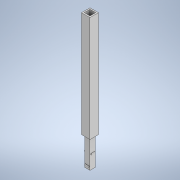
# Autodesk Inventor part: Część1
Saved by Autodesk Inventor 2022 (Build 260153000, 153)
## iProperties
Created: 2022-10-22
Part Number: Część1
Material: Ogólny
Document SubType Name: Modeling
Designer: kosak
Density: 1 g/cm^3
Appearance: Domyślna
Author: kosak
Autodesk Inventor part; units mm, degrees
ref_plane "YZ Plane" through (0, 0, 0) normal (1, 0, 0) x (0, 1, 0)
ref_plane "XZ Plane" through (0, 0, 0) normal (0, 1, 0) x (-1, 0, 0)
ref_plane "XY Plane" through (0, 0, 0) normal (0, 0, 1) x (1, 0, 0)
sketch "Szkic1" plane through (0, 0, 0) normal (0, 1, 0) x (-1, 0, 0)
  line L0 (0, 0) -> (12, 0)
  line L1 (12, 0) -> (12, -12)
  line L2 (12, -12) -> (0, -12)
  line L3 (0, -12) -> (0, 0)
  dimension "d0" = 12
  dimension "d1" = 12
  constraints: 8 end point, 2 parallel, 1 horizontal, 1 perpendicular
  measures "d0" distance of L1.end L2.end
  measures "d1" distance of L0.end L1.end
extrude "Wyciągnięcie proste1" add sketch "Szkic1" along normal blind 86
sketch "Szkic2" plane through (0, 86, 0) normal (0, 1, 0) x (1, 0, 0)
  line L0 (0, 12) -> (-12, 12) projected
  line L1 (-12, 12) -> (-12, 0) projected
  line L2 (-12, 0) -> (0, 0) projected
  line L3 (0, 0) -> (0, 12) projected
  line L4 (-10, 2) -> (-10, 10)
  line L5 (-10, 10) -> (-2, 10)
  line L6 (-2, 10) -> (-2, 2)
  line L7 (-2, 2) -> (-10, 2)
  dimension "d4" = 2
  constraints: 8 end point, 3 other
  measures "d4" distance between parallel lines of L1 L4
extrude "Wyciągnięcie proste2" cut sketch "Szkic2" against normal blind 86 contours L4 L5 L6 L7
sketch "Szkic9" plane through (0, 0, 0) normal (0, -1, 0) x (1, 0, 0)
  line L0 (-2, -10) -> (-10, -10) projected
  line L1 (-2, -2) -> (-2, -10) projected
  line L2 (-10, -2) -> (-2, -2) projected
  line L3 (-10, -10) -> (-10, -2) projected
  line L4 (-2.3, -2.3) -> (-2.3, -9.7)
  line L5 (-2.3, -9.7) -> (-9.7, -9.7)
  line L6 (-9.7, -9.7) -> (-9.7, -2.3)
  line L7 (-9.7, -2.3) -> (-2.3, -2.3)
  line L8 (-3.3, -3.3) -> (-3.3, -8.7)
  line L9 (-3.3, -8.7) -> (-8.7, -8.7)
  line L10 (-8.7, -8.7) -> (-8.7, -3.3)
  line L11 (-8.7, -3.3) -> (-3.3, -3.3)
  point P0 (0, 0)
  dimension "d21" = 0.3
  dimension "d22" = 1
  constraints: 16 end point, 6 other
  measures "d21" distance between parallel lines of L2 L7
  measures "d22" distance between parallel lines of L7 L11
extrude "Wyciągnięcie proste8" add sketch "Szkic9" along normal blind 40 contours L4 L5 L6 L7
sketch "Szkic10" plane through (0, 0, 0) normal (0, 1, 0) x (1, 0, 0)
  line L0 (-2, 2) -> (-2, 10) projected
  line L1 (-10.1182, 1.9087) -> (-2, 1.9087)
  line L2 (-2, 1.9087) -> (-2, 10)
  line L3 (-2, 10) -> (-10.1182, 10)
  line L4 (-10.1182, 10) -> (-10.1182, 1.9087)
  line L5 (-3.3, 3.3) -> (-3.3, 8.7) projected
  line L6 (-8.7, 3.3) -> (-3.3, 3.3) projected
  line L7 (-8.7, 8.7) -> (-8.7, 3.3) projected
  line L8 (-3.3, 8.7) -> (-8.7, 8.7) projected
  line L9 (-8.7, 3.3) -> (-3.3, 3.3)
  line L10 (-3.3, 3.3) -> (-3.3, 8.7)
  line L11 (-3.3, 8.7) -> (-8.7, 8.7)
  line L12 (-8.7, 8.7) -> (-8.7, 3.3)
  point P0 (0, 0)
  constraints: 16 end point, 4 parallel, 2 horizontal, 2 perpendicular
extrude "Wyciągnięcie proste9" add sketch "Szkic10" along normal blind 2
sketch "Szkic11" plane through (-9.7, 0, -9.7) normal (-1, 0, 0) x (0, 0, 1)
  line L0 (7.4, 0) -> (0, 0) projected
  line L1 (2.1159, 0) -> (2.1159, -20)
  line L2 (1, 2) -> (1, -40) projected
  line L3 (6.4, 2) -> (6.4, -40) projected
  line L4 (1, -20) -> (6.4, -20)
  line L5 (6.4, -20) -> (6.4, -21.6)
  line L6 (6.4, -21.6) -> (1, -21.6)
  line L7 (1, -21.6) -> (1, -20)
  point P0 (9.7, 0)
  point P1 (1, -21.6)
  dimension "d27" = 20
  dimension "d28" = 1.6
  constraints: 10 end point, 3 point on line, 2 parallel, 1 horizontal, 1 perpendicular, 1 vertical
  measures "d27" distance of L1.start L1.end
  measures "d28" distance of L4.end L5.end
extrude "Wyciągnięcie proste10" add sketch "Szkic11" along normal blind 1.4 contours L3 L6 L2 L4
pattern_linear "Szyk prostokątny1" count 2 spacing 8.4 along (1, 0, 0) of "Wyciągnięcie proste10"
sketch "Szkic12" plane through (-9.7, 0, -2.3) normal (0, 0, 1) x (1, 0, 0)
  line L0 (9.7, 0) -> (-2.3, 0) projected
  line L1 (2.9125, 0) -> (2.9125, -35)
  line L2 (1, 2) -> (1, -40) projected
  line L3 (1, 2) -> (1, -40) projected
  line L4 (6.4, 2) -> (6.4, -40) projected
  line L5 (1, -35) -> (6.4, -35)
  line L6 (6.4, -35) -> (6.4, -36.6)
  line L7 (6.4, -36.6) -> (1, -36.6)
  line L8 (1, -36.6) -> (1, -35)
  dimension "d34" = 35
  dimension "d35" = 1.6
  constraints: 10 end point, 3 parallel, 3 point on line, 1 horizontal, 1 perpendicular
  measures "d34" distance of L1.start L1.end
  measures "d35" distance of L5.end L6.end
extrude "Wyciągnięcie proste11" add sketch "Szkic12" along normal blind 1.4 contours L4 L7 L2 L5
pattern_linear "Szyk prostokątny2" count 2 spacing 8.4 along (0, 0, -1) of "Wyciągnięcie proste11"
fillet "Zaokrąglenie1" radius 2 4 edges at (-8.7, 2, -6) (-6, 2, -3.3) (-6, 2, -8.7) (-3.3, 2, -6)
sketch "Szkic13" plane through (0, 86, 0) normal (0, 1, 0) x (1, 0, 0)
  line L0 (0, 0) -> (0, 12) projected
  line L1 (-12, 12) -> (-12, 0) projected
  line L2 (0, 0) -> (-12, 0)
  line L3 (-12, 0) -> (-12, 12)
  line L4 (-12, 12) -> (0, 12)
  line L5 (0, 12) -> (0, 0)
  line L6 (-2, 10) -> (-2, 2) projected
  line L7 (-10, 2) -> (-10, 10) projected
  line L8 (-2, 2) -> (-10, 2)
  line L9 (-10, 2) -> (-10, 10)
  line L10 (-10, 10) -> (-2, 10)
  line L11 (-2, 10) -> (-2, 2)
  constraints: 16 end point, 4 parallel, 2 horizontal, 2 perpendicular
extrude "Wyciągnięcie proste12" add sketch "Szkic13" along normal blind 63
fillet "Zaokrąglenie2" radius 0.8 8 edges at (-11.1, -20, -6) (-11.1, -21.6, -6) (-1.3, -20, -6) (-1.3, -21.6, -6) (-6, -36.6, -0.9) (-6, -35, -0.9) (-6, -35, -10.7) (-6, -36.6, -10.7)
